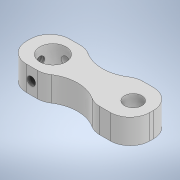
# Autodesk Inventor part: Tube to TRB1 adapter
Saved by Autodesk Inventor 2021.2 (Build 252289000, 289)
## iProperties
Created: 2021-07-01
Part Number: Tube to TRB1 adapter
Material: Generic
Document SubType Name: Modeling
Designer: jl4459
Density: 1 g/cm^3
Appearance: Default
Author: jl4459
Autodesk Inventor part; units mm, degrees
note: some values were not read from the file. Chosen so that the rebuilt part matches the saved one: direction of "Hole4".
ref_plane "YZ Plane" through (0, 0, 0) normal (1, 0, 0) x (0, 1, 0)
ref_plane "XZ Plane" through (0, 0, 0) normal (0, 1, 0) x (-1, 0, 0)
ref_plane "XY Plane" through (0, 0, 0) normal (0, 0, 1) x (1, 0, 0)
sketch "Sketch1" plane through (0, 0, 0) normal (0, 1, 0) x (-1, 0, 0)
  line L0 (15.875, 5.5563) -> (-15.875, 5.5563)
  line L1 (-15.875, 5.5563) -> (-15.875, -5.5563)
  line L2 (-15.875, -5.5563) -> (15.875, -5.5563)
  line L3 (15.875, -5.5563) -> (15.875, 5.5563)
  point P0 (0, 0)
  dimension "d0" = 31.75
  dimension "d1" = 11.1125
  constraints: 8 end point, 2 parallel, 1 horizontal, 1 perpendicular
  measures "d0" distance of L2.end L1.end
  measures "d1" distance of L1.end L0.end
extrude "Extrusion1" add sketch "Sketch1" along normal blind 6.35
sketch "Sketch2" plane through (0, 6.35, 0) normal (0, 1, 0) x (1, 0, 0)
  line L0 (15.875, -5.5563) -> (15.875, 5.5563) projected
  line L1 (15.875, 5.5563) -> (-15.875, 5.5563) projected
  point P0 (0, 0)
  point P1 (11.1125, 0)
  dimension "d4" = 4.7625
  dimension "d5" = 5.5563
  measures "d4" distance from line of L0 point (11.112, 0)
  measures "d5" distance from line of L1 point (11.112, 0)
hole "Hole1" at (11.1125, 6.35, 0) direction (0, -1, 0) diameter 4.4958 end through all clearance for "Flat Head Machine Screw (82)" size "#8" standard "Ansi Unified Screw Threads"
sketch "Sketch3" plane through (0, 6.35, 0) normal (0, 1, 0) x (1, 0, 0)
  line L0 (-15.875, 5.5563) -> (-15.875, -5.5563) projected
  line L1 (15.875, 5.5563) -> (-15.875, 5.5563) projected
  point P0 (0, 0)
  point P1 (-9.525, 0)
  dimension "d13" = 6.35
  dimension "d14" = 5.5563
  measures "d13" distance from line of L0 point (-9.525, 0)
  measures "d14" distance from line of L1 point (-9.525, 0)
hole "Hole2" at (-9.525, 6.35, 0) direction (0, -1, 0) diameter 6.7564 end through all clearance for "Flat Head Machine Screw (82)" size "1/4" standard "Ansi Unified Screw Threads"
fillet "Fillet1" radius 5.08 4 edges at (15.875, 3.175, -5.5563) (15.875, 3.175, 5.5563) (-15.875, 3.175, -5.5563) (-15.875, 3.175, 5.5563)
sketch "Sketch4" plane through (0, 6.35, 0) normal (0, 1, 0) x (1, 0, 0)
  line L0 (-10.795, -5.5563) -> (10.795, -5.5563) projected
  arc A0 (6.35, -5.5563) -> (-6.35, -5.5563) centre (0, -12.8323) ccw
  line L1 (10.795, 5.5563) -> (-10.795, 5.5563) projected
  arc A1 (-6.35, 5.5563) -> (6.35, 5.5563) centre (0, 12.8323) ccw
  point P0 (0, 0)
  dimension "d23" = 12.7
  dimension "d24" = 12.7
  constraints: 4 point on circle, 4 point on line, 2 centre point
  measures "d23" distance of A0.start A0.end
  measures "d24" distance of A1.end A1.start
extrude "Extrusion2" cut sketch "Sketch4" against normal blind 6.35
fillet "Fillet2" radius 5.08 4 edges at (-6.35, 3.175, -5.5563) (6.35, 3.175, -5.5563) (-6.35, 3.175, 5.5563) (6.35, 3.175, 5.5563)
sketch "Sketch5" plane through (-10.795, 0, 5.5563) normal (0, 0, 1) x (1, 0, 0)
  line L0 (0, 6.35) -> (2.7628, 6.35) projected
  line L1 (-5.08, 6.35) -> (-5.08, 0) projected
  point P0 (10.795, 0)
  point P1 (1.27, 3.175)
  dimension "d28" = 3.175
  dimension "d29" = 6.35
  measures "d28" distance from line of L0 point (1.27, 3.175)
  measures "d29" distance from line of L1 point (1.27, 3.175)
hole "Hole3" at (-9.525, 3.175, 5.5563) direction (0, 0, -1) diameter 2.1565 end through all thread size "4-40 UNC" class "2B" standard "ANSI Unified Screw Threads"
sketch "Sketch6" plane through (-15.875, 0, -0.4763) normal (-1, 0, 0) x (0, 0, 1)
  line L0 (0, 6.35) -> (0.9525, 6.35) projected
  line L1 (-5.08, 6.35) -> (-5.08, 0) projected
  point P0 (0.4763, 0)
  point P1 (0.4474, 3.175)
  dimension "d37" = 3.175
  dimension "d38" = 5.5274
  measures "d37" distance from line of L0 point (0.447, 3.175)
  measures "d38" distance from line of L1 point (0.447, 3.175)
hole "Hole4" at (-15.875, 3.175, -0.0288) direction (1, 0, 0) diameter 2.1565 end up to surface thread size "4-40 UNC" class "2B" standard "ANSI Unified Screw Threads"
body "Solid1"
